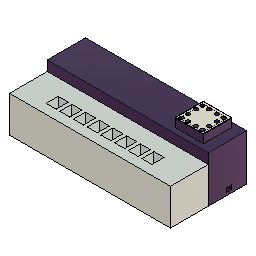
CAD File (2) (Autodesk Fusion 360 design; units mm, degrees)
Autodesk Fusion 360 part; units mm, degrees
sketch "Sketch1" plane through (0, 0, 0) normal (0, 0, 1) x (1, 0, 0)
sketch "Sketch2" plane through (0, 0, 0) normal (0, 0, 1) x (1, 0, 0)
  line L0 (0, 0) -> (-40, 0)
  line L1 (-40, 0) -> (-40, -9.5)
  line L2 (-40, -9.5) -> (0, -9.5)
  line L3 (0, -9.5) -> (0, 0)
  dimension "d1" = 40
  dimension "d2" = 9.5
  constraint horizontal L0
  constraint vertical L1
  constraint horizontal L2
  constraint vertical L3
  constraint coincident L0.start L3.end
  measures "d1" distance of L0.start L0.end
  measures "d2" distance of L0.end L1.end
extrude "Extrude1" add sketch "Sketch2" along normal blind 11.5 makes body 1
sketch "Sketch3" plane through (0, 0, 0) normal (0, 0, 1) x (1, 0, 0)
  line L0 (-39.9718, -9.6631) -> (0.0282, -9.6631)
  line L1 (0.0282, -9.6631) -> (0.0282, -19.0631)
  line L2 (0.0282, -19.0631) -> (-39.9718, -19.0631)
  line L3 (-39.9718, -19.0631) -> (-39.9718, -9.6631)
  dimension "d5" = 40
  dimension "d6" = 9.4
  constraint horizontal L0
  constraint vertical L1
  constraint horizontal L2
  constraint vertical L3
  measures "d5" distance of L1.end L2.end
  measures "d6" distance of L0.start L2.end
extrude "Extrude2" add sketch "Sketch3" along normal blind 9 separate body makes body 2
move_body "Move1" bodies 2 to x (1, 0, 0) y (0, 1, 0) z (0, 0, 1) at (0, 0.163, 0)
move_body "Move2" bodies 2 to x (1, 0, 0) y (0, 1, 0) z (0, 0, 1) at (0, 0, 0.028)
move_body "Move3" bodies 2 to x (1, 0, 0) y (0, 1, 0) z (0, 0, 1) at (0.028, 0, 0)
move_body "Move4" bodies 2 to x (1, 0, 0) y (0, 1, 0) z (0, 0, 1) at (-0.056, 0, 0)
move_body "Move5" bodies 2 to x (1, 0, 0) y (0, 1, 0) z (0, 0, 1) at (0, 0, -0.028)
sketch "Sketch4" plane through (0, 0, 0) normal (0, 0, 1) x (1, 0, 0)
  line L0 (-17.2004, -16.5, 9) -> (-19.7004, -16.5, 9)
  line L1 (-19.7004, -16.5, 9) -> (-19.7004, -13.5, 9)
  line L2 (-19.7004, -13.5, 9) -> (-17.2004, -13.5, 9)
  line L3 (-17.2004, -13.5, 9) -> (-17.2004, -16.5, 9)
  line L4 (-23.1004, -13.5, 9) -> (-20.6004, -13.5, 9)
  line L5 (-20.6004, -13.5, 9) -> (-20.6004, -16.5, 9)
  line L6 (-20.6004, -16.5, 9) -> (-23.1004, -16.5, 9)
  line L7 (-23.1004, -16.5, 9) -> (-23.1004, -13.5, 9)
  line L8 (-24.0004, -16.5, 9) -> (-26.5004, -16.5, 9)
  line L9 (-26.5004, -16.5, 9) -> (-26.5004, -13.5, 9)
  line L10 (-26.5004, -13.5, 9) -> (-24.0004, -13.5, 9)
  line L11 (-24.0004, -13.5, 9) -> (-24.0004, -16.5, 9)
  line L12 (-27.4004, -16.5, 9) -> (-29.9004, -16.5, 9)
  line L13 (-29.9004, -16.5, 9) -> (-29.9004, -13.5, 9)
  line L14 (-29.9004, -13.5, 9) -> (-27.4004, -13.5, 9)
  line L15 (-27.4004, -13.5, 9) -> (-27.4004, -16.5, 9)
  line L16 (-30.8004, -16.5, 9) -> (-33.3004, -16.5, 9)
  line L17 (-33.3004, -16.5, 9) -> (-33.3004, -13.5, 9)
  line L18 (-33.3004, -13.5, 9) -> (-30.8004, -13.5, 9)
  line L19 (-30.8004, -13.5, 9) -> (-30.8004, -16.5, 9)
  line L20 (-40, -9.5) -> (0, -9.5)
  line L21 (-16.3004, -13.5, 9) -> (-13.8004, -13.5, 9)
  line L22 (-13.8004, -13.5, 9) -> (-13.8004, -16.5, 9)
  line L23 (-13.8004, -16.5, 9) -> (-16.3004, -16.5, 9)
  line L24 (-16.3004, -16.5, 9) -> (-16.3004, -13.5, 9)
  line L25 (-12.9004, -13.5, 9) -> (-10.4004, -13.5, 9)
  line L26 (-10.4004, -13.5, 9) -> (-10.4004, -16.5, 9)
  line L27 (-10.4004, -16.5, 9) -> (-12.9004, -16.5, 9)
  line L28 (-12.9004, -16.5, 9) -> (-12.9004, -13.5, 9)
  line L29 (-9.5004, -13.5, 9) -> (-7.0004, -13.5, 9)
  line L30 (-7.0004, -13.5, 9) -> (-7.0004, -16.5, 9)
  line L31 (-7.0004, -16.5, 9) -> (-9.5004, -16.5, 9)
  line L32 (-9.5004, -16.5, 9) -> (-9.5004, -13.5, 9)
sketch "Sketch5" plane through (0, 0, 9) normal (0, 0, 1) x (-1, 0, 0)
  line L0 (39.9998, 18.9001) -> (-0.0002, 18.9001)
  line L1 (-0.0002, 18.9001) -> (-0.0002, 9.5001)
  line L2 (-0.0002, 9.5001) -> (39.9998, 9.5001)
  line L3 (39.9998, 9.5001) -> (39.9998, 18.9001)
extrude "Extrude3" cut sketch "Sketch4" against normal blind 6 contours L0 L1 L2 L3 | L4 L5 L6 L7 | L8 L9 L10 L11 | L12 L13 L14 L15 | L16 L17 L18 L19 | L21 L22 L23 L24 | L25 L26 L27 L28 | L29 L30 L31 L32 in plane through (0, 0, 9) normal (0, 0, 1) bodies 2
sketch "Sketch6" plane through (0, 0, 11.5) normal (0, 0, 1) x (-1, 0, 0)
  line L0 (0, 9.5) -> (0, 0)
  line L1 (0, 0) -> (40, 0)
  line L2 (40, 0) -> (40, 9.5)
  line L3 (40, 9.5) -> (0, 9.5)
fillet "Fillet1" radius 0.1 1 edges at (-40, 0, 5.75) on bodies 1
sketch "Sketch7" plane through (0, 0, 0) normal (0, 0, 1) x (1, 0, 0)
  line L0 (-9.5546, -1.1433, 11.5) -> (-2.5546, -1.1433, 11.5)
  line L1 (-2.5546, -1.1433, 11.5) -> (-2.5546, -8.1433, 11.5)
  line L2 (-2.5546, -8.1433, 11.5) -> (-9.5546, -8.1433, 11.5)
  line L3 (-9.5546, -8.1433, 11.5) -> (-9.5546, -1.1433, 11.5)
extrude "Extrude4" add sketch "Sketch7" along normal blind 2 contours L0 L1 L2 L3 in plane through (0, 0, 11.5) normal (0, 0, 1) bodies 1
sketch "Sketch8" plane through (0, 0, 0) normal (1, 0, 0) x (0, 1, 0)
  line L0 (-4.9523, 1.6508) -> (-3.6824, 1.6508)
  line L1 (-3.6824, 1.6508) -> (-3.6824, 0.7619)
  line L2 (-3.6824, 0.7619) -> (-4.9523, 0.7619)
  line L3 (-4.9523, 0.7619) -> (-4.9523, 1.6508)
  constraint horizontal L0
  constraint vertical L1
  constraint horizontal L2
  constraint vertical L3
extrude "Extrude5" cut sketch "Sketch8" against normal blind 4 bodies 1
sketch "Sketch9" plane through (0, 0, 13.5) normal (0, 0, 1) x (-1, 0, 0)
  line L0 (9.5546, 8.1433) -> (2.5546, 8.1433)
  line L1 (2.5546, 8.1433) -> (2.5546, 1.1433)
  line L2 (2.5546, 1.1433) -> (9.5546, 1.1433)
  line L3 (9.5546, 1.1433) -> (9.5546, 8.1433)
  line L4 (3.0546, 7.6433) -> (9.0546, 7.6433)
  line L5 (9.0546, 7.6433) -> (9.0546, 1.6433)
  line L6 (9.0546, 1.6433) -> (3.0546, 1.6433)
  line L7 (3.0546, 1.6433) -> (3.0546, 7.6433)
  dimension "d69" = 0.5
  dimension "d70" = 0.5
  dimension "d71" = 0.5
  dimension "d72" = 0.5
  constraint horizontal L4
  constraint vertical L5
  constraint horizontal L6
  constraint vertical L7
  measures "d69" distance of L0 L4
  measures "d70" distance of L1 L7
  measures "d71" distance of L2 L6
  measures "d72" distance of L3 L5
extrude "Extrude6" cut sketch "Sketch9" against normal blind 2 contours L4 L5 L6 L7 bodies 1
sketch "Sketch10" plane through (0, 0, 0) normal (0, 0, 1) x (1, 0, 0)
  line L0 (-2.6198, -8.1119, 13.6232) -> (-9.5917, -8.1119, 13.6232)
  line L1 (-9.5917, -8.1119, 13.6232) -> (-9.5917, -1.14, 13.6232)
  line L2 (-9.5917, -1.14, 13.6232) -> (-2.6198, -1.14, 13.6232)
  line L3 (-2.6198, -1.14, 13.6232) -> (-2.6198, -8.1119, 13.6232)
  line L4 (0, 0) -> (-40, 0)
extrude "Extrude7" add sketch "Sketch10" along normal blind 0.001 separate body contours L0 L1 L2 L3 in plane through (0, 0, 13.6232) normal (0, 0, 1) makes body 3
sketch "Sketch12" plane through (0, 0, 13.6242) normal (0, 0, 1) x (-1, 0, 0)
  line L0 (2.6198, 1.14) -> (9.5917, 1.14)
  line L1 (9.5917, 1.14) -> (9.5917, 8.1119)
  line L2 (9.5917, 8.1119) -> (2.6198, 8.1119)
  line L3 (2.6198, 8.1119) -> (2.6198, 1.14)
  circle A0 centre (3.5407, 7.3433) radius 0.5
  circle A1 centre (3.5402, 2.1809) radius 0.5
  circle A2 centre (8.7402, 2.1811) radius 0.5
  circle A3 centre (8.7405, 7.3811) radius 0.5
  circle A4 centre (7.1405, 7.3811) radius 0.5
  circle A5 centre (5.1407, 7.3811) radius 0.5
  circle A6 centre (3.5407, 5.7433) radius 0.5
  circle A7 centre (3.5407, 3.7809) radius 0.5
  circle A8 centre (5.1402, 2.1809) radius 0.5
  circle A9 centre (7.1402, 2.1809) radius 0.5
  circle A10 centre (8.7402, 3.7811) radius 0.5
  circle A11 centre (8.7402, 5.7811) radius 0.5
  dimension "d131" = 1
  dimension "d132" = 1
  dimension "d133" = 1
  dimension "d134" = 1
  dimension "d135" = 1
  dimension "d136" = 1
  dimension "d137" = 1
  dimension "d138" = 1
  dimension "d139" = 1
  dimension "d140" = 1
  dimension "d141" = 1
  dimension "d142" = 1
  dimension "d143" = 1.6
  dimension "d144" = 1.9998
  dimension "d145" = 1.6
  dimension "d146" = 1.6
  dimension "d147" = 2
  dimension "d148" = 1.6
  dimension "d149" = 5.9309
  dimension "d150" = 5.931
  dimension "d151" = 5.931
  dimension "d152" = 5.931
  dimension "d153" = 1.6
  dimension "d154" = 2
  dimension "d155" = 1.6
  dimension "d156" = 6.0515
  dimension "d157" = 6.051
  dimension "d158" = 6.051
  dimension "d159" = 6.051
  dimension "d160" = 1.6
  dimension "d161" = 1.6
  measures "d131" diameter of A5
  measures "d132" diameter of A4
  measures "d133" diameter of A3
  measures "d134" diameter of A0
  measures "d135" diameter of A6
  measures "d136" diameter of A7
  measures "d137" diameter of A1
  measures "d138" diameter of A8
  measures "d139" diameter of A9
  measures "d140" diameter of A2
  measures "d141" diameter of A10
  measures "d142" diameter of A11
  measures "d143" horizontal distance of A0.centre A5.centre
  measures "d144" distance of A4.centre A5.centre
  measures "d145" distance of A3.centre A4.centre
  measures "d146" vertical distance of A3.centre A11.centre
  measures "d147" distance of A10.centre A11.centre
  measures "d148" distance of A2.centre A10.centre
  measures "d149" distance of L2 A2.centre
  measures "d150" distance of L2 A9.centre
  measures "d151" distance of L2 A8.centre
  measures "d152" distance of L2 A1.centre
  measures "d153" horizontal distance of A2.centre A9.centre
  measures "d154" distance of A8.centre A9.centre
  measures "d155" distance of A1.centre A8.centre
  measures "d156" distance of L1 A1.centre
  measures "d157" distance of L1 A7.centre
  measures "d158" distance of L1 A6.centre
  measures "d159" distance of L1 A0.centre
  measures "d160" distance of A0.centre A6.centre
  measures "d161" vertical distance of A1.centre A7.centre
extrude "Extrude8" cut sketch "Sketch12" against normal blind 0.5 contours A0 | A1 | A2 | A3 | A4 | A5 | A6 | A7 | A8 | A9 | A10 | A11 bodies 1 3
